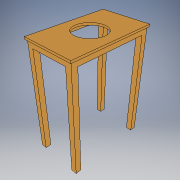
# Autodesk Inventor part: table
Saved by Autodesk Inventor 2018 (Build 220112000, 112)
## iProperties
Created: 2018-10-18
Part Number: table
Material: Laminated Veneer Lumber
Document SubType Name: Modeling
Designer: freyja
Density: 0.51 g/cm^3
Appearance: Plywood - New
Author: freyja
Autodesk Inventor part; units mm, degrees
ref_plane "YZ Plane" through (0, 0, 0) normal (1, 0, 0) x (0, 1, 0)
ref_plane "XZ Plane" through (0, 0, 0) normal (0, 1, 0) x (-1, 0, 0)
ref_plane "XY Plane" through (0, 0, 0) normal (0, 0, 1) x (1, 0, 0)
sketch "Sketch1" plane through (0, 0, 0) normal (0, 1, 0) x (-1, 0, 0)
  line L0 (457.2, 762) -> (-457.2, 762)
  line L1 (-457.2, 762) -> (-457.2, -762)
  line L2 (-457.2, -762) -> (457.2, -762)
  line L3 (457.2, -762) -> (457.2, 762)
  line L4 (457.2, 762) -> (-457.2, -762) construction
  line L5 (-457.2, 762) -> (457.2, -762) construction
  point P0 (0, 0)
  dimension "d0" = 914.4
  dimension "d1" = 1524
  constraints: 12 end point, 2 midpoint, 2 parallel, 1 horizontal, 1 perpendicular
  measures "d0" distance of L2.end L1.end
  measures "d1" distance of L1.end L0.end
extrude "Extrusion1" add sketch "Sketch1" along normal blind 38.1
sketch "Sketch2" plane through (0, 0, 0) normal (0, -1, 0) x (1, 0, 0)
  line L0 (-381, 685.8) -> (381, 685.8) construction
  line L1 (381, 685.8) -> (381, -685.8) construction
  line L2 (381, -685.8) -> (-381, -685.8) construction
  line L3 (-381, -685.8) -> (-381, 685.8) construction
  line L4 (-381, 685.8) -> (381, -685.8) construction
  line L5 (381, 685.8) -> (-381, -685.8) construction
  line L6 (330.2, 736.6) -> (431.8, 736.6)
  line L7 (431.8, 736.6) -> (431.8, 635)
  line L8 (431.8, 635) -> (330.2, 635)
  line L9 (330.2, 635) -> (330.2, 736.6)
  line L10 (330.2, 736.6) -> (431.8, 635) construction
  line L11 (431.8, 736.6) -> (330.2, 635) construction
  line L12 (431.8, -635) -> (330.2, -635)
  line L13 (330.2, -635) -> (330.2, -736.6)
  line L14 (330.2, -736.6) -> (431.8, -736.6)
  line L15 (431.8, -736.6) -> (431.8, -635)
  line L16 (431.8, -635) -> (330.2, -736.6) construction
  line L17 (330.2, -635) -> (431.8, -736.6) construction
  line L18 (-431.8, -736.6) -> (-330.2, -736.6)
  line L19 (-330.2, -736.6) -> (-330.2, -635)
  line L20 (-330.2, -635) -> (-431.8, -635)
  line L21 (-431.8, -635) -> (-431.8, -736.6)
  line L22 (-431.8, -736.6) -> (-330.2, -635) construction
  line L23 (-330.2, -736.6) -> (-431.8, -635) construction
  line L24 (-431.8, 736.6) -> (-330.2, 736.6)
  line L25 (-330.2, 736.6) -> (-330.2, 635)
  line L26 (-330.2, 635) -> (-431.8, 635)
  line L27 (-431.8, 635) -> (-431.8, 736.6)
  line L28 (-431.8, 736.6) -> (-330.2, 635) construction
  line L29 (-330.2, 736.6) -> (-431.8, 635) construction
  point P0 (0, 0)
  dimension "d6" = 762
  dimension "d7" = 1371.6
  dimension "d8" = 101.6
  dimension "d9" = 101.6
  dimension "d10" = 101.6
  dimension "d11" = 101.6
  dimension "d12" = 101.6
  dimension "d13" = 101.6
  dimension "d14" = 101.6
  dimension "d15" = 101.6
  constraints: 60 end point, 10 midpoint, 10 parallel, 5 horizontal, 5 perpendicular
  measures "d6" distance of L1.end L2.end
  measures "d7" distance of L0.end L1.end
  measures "d8" distance of L7.end L8.end
  measures "d9" distance of L6.end L7.end
  measures "d10" distance of L14.end L13.end
  measures "d11" distance of L13.end L12.end
  measures "d12" distance of L20.end L19.end
  measures "d13" distance of L19.end L18.end
  measures "d14" distance of L25.end L26.end
  measures "d15" distance of L24.end L25.end
extrude "Extrusion2" add sketch "Sketch2" along normal blind 1981.2
sketch "Sketch3" plane through (0, 0, 0) normal (0, -1, 0) x (1, 0, 0)
  line L0 (431.8, 635) -> (330.2, 635) projected
  line L1 (431.8, 635) -> (381, 635)
  line L2 (381, 635) -> (381, -635)
  line L3 (381, -635) -> (431.8, -635)
  line L4 (431.8, -635) -> (431.8, 635)
  line L5 (0, 0) -> (0, -69.3079) construction
  line L6 (-431.8, 635) -> (-330.2, 635)
  line L7 (-431.8, 635) -> (-381, 635)
  line L8 (-381, 635) -> (-381, -635)
  line L9 (-381, -635) -> (-431.8, -635)
  line L10 (-431.8, -635) -> (-431.8, 635)
  line L11 (330.2, -736.6) -> (330.2, -635) projected
  line L12 (-330.2, -736.6) -> (330.2, -736.6)
  line L13 (330.2, -736.6) -> (330.2, -685.8)
  line L14 (330.2, -685.8) -> (-330.2, -685.8)
  line L15 (-330.2, -685.8) -> (-330.2, -736.6)
  line L16 (0, 0) -> (54.1332, 0) construction
  line L17 (330.2, 736.6) -> (330.2, 635)
  line L18 (-330.2, 736.6) -> (330.2, 736.6)
  line L19 (330.2, 736.6) -> (330.2, 685.8)
  line L20 (330.2, 685.8) -> (-330.2, 685.8)
  line L21 (-330.2, 685.8) -> (-330.2, 736.6)
  dimension "d18" = 50.8
  dimension "d19" = 1270
  dimension "d20" = 50.8
  constraints: 40 end point, 10 symmetric about line, 4 parallel, 3 horizontal, 2 perpendicular, 1 midpoint, 1 vertical
  measures "d18" distance of L3.end L2.end
  measures "d19" distance of L2.end L1.end
  measures "d20" distance of L13.end L12.end
extrude "Extrusion3" add sketch "Sketch3" along normal blind 101.6
sketch "Sketch4" plane through (0, 38.1, 0) normal (0, 1, 0) x (1, 0, 0)
  circle A0 centre (0, 0) radius 279.4
  dimension "d23" = 558.8
  constraints: 1 centre point, 1 coincident
  measures "d23" diameter of A0
extrude "Extrusion4" cut sketch "Sketch4" against normal blind 101.6
body "Solid1"
